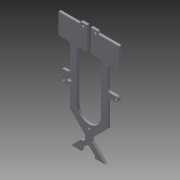
# Autodesk Inventor part: dissipador curvas 2mm v2
Saved by Autodesk Inventor 2013 (Build 170138000, 138)
## iProperties
Created: 2015-01-15
Part Number: dissipador curvas 2mm v2
Material: Genérico
Document SubType Name: Modeling
Designer: fernando.santanna
Density: 1 g/cm^3
Author: fernando.santanna
Autodesk Inventor part; units mm, degrees
ref_plane "YZ Plane" through (0, 0, 0) normal (1, 0, 0) x (0, 1, 0)
ref_plane "XZ Plane" through (0, 0, 0) normal (0, 1, 0) x (-1, 0, 0)
sketch "Bloco2" plane through (0, 0, 0) normal (0, 0, 1) x (1, 0, 0)
  line L0 (61.8192, 99.9321) -> (61.8192, 104.9321) construction
  line L1 (61.8192, 104.9321) -> (61.8192, 99.9321)
  line L2 (57.3192, 104.9321) -> (58.3192, 104.9321)
  line L3 (58.3192, 104.9321) -> (58.3192, 99.9321)
  line L4 (58.3192, 99.9321) -> (57.3192, 99.9321)
  line L5 (57.3192, 99.9321) -> (57.3192, 104.9321)
  line L6 (65.3192, 104.9321) -> (66.3192, 104.9321)
  line L7 (66.3192, 104.9321) -> (66.3192, 99.9321)
  line L8 (66.3192, 99.9321) -> (65.3192, 99.9321)
  line L9 (65.3192, 99.9321) -> (65.3192, 104.9321)
  point P0 (61.8192, 102.4321)
  dimension "d1" = 1
  dimension "d3" = 3.5
  dimension "d4" = 5
  dimension "d5" = 1
  dimension "d6" = 5
  dimension "d7" = 3.5
  measures "d1" distance of L3.end L4.end
  measures "d3" distance between parallel lines of L0 L3
  measures "d4" distance of L4.end L2.start
  measures "d5" distance of L7.end L8.end
  measures "d6" distance of L6.end L7.end
  measures "d7" distance between parallel lines of L1 L9
sketch "Bloco1" plane through (0, 0, 0) normal (0, 0, 1) x (1, 0, 0)
  arc A0 (51.7292, 104.9321) -> (48.7292, 101.9321) centre (51.7292, 101.9321) ccw construction
  arc A1 (93.7292, 2.9321) -> (91.7292, 4.9321) centre (91.7292, 2.9321) ccw construction
  line L0 (64.3092, -0.0679) -> (64.3092, 4.9321) construction
  circle A2 centre (73.7292, 25.9321) radius 1.1 construction
  circle A3 centre (51.5292, 57.9321) radius 1.1 construction
  circle A4 centre (94.7292, 50.4321) radius 1.1 construction
  circle A5 centre (56.5292, 2.9321) radius 1.1 construction
  circle A6 centre (68.7292, 96.9321) radius 1.1 construction
  circle A7 centre (91.7292, 2.9321) radius 1.1 construction
  circle A8 centre (78.7292, 96.9321) radius 1.1 construction
  arc A9 (91.2292, 48.4321) -> (89.2292, 46.4321) centre (91.2292, 46.4321) ccw construction
  line L1 (91.2292, 48.4321) -> (94.7807, 48.4321) construction
  arc A10 (94.7292, 48.4321) -> (96.7292, 50.4321) centre (94.7292, 50.4321) ccw construction
  line L2 (96.7292, 50.3807) -> (96.7292, 53.9321) construction
  arc A11 (91.1261, 55.1256) -> (90.851, 51.4175) centre (90.2532, 53.3261) ccw construction
  arc A12 (96.7292, 53.9321) -> (94.7292, 55.9321) centre (94.7292, 53.9321) ccw construction
  line L3 (91.2292, 55.9321) -> (94.7292, 55.9321) construction
  arc A13 (89.2292, 57.9321) -> (91.2292, 55.9321) centre (91.2292, 57.9321) ccw construction
  line L4 (83.7292, 38.9321) -> (83.7292, 77.9321) construction
  arc A14 (83.7292, 77.9321) -> (81.7292, 79.9321) centre (81.7292, 77.9321) ccw construction
  line L5 (77.2292, 79.9321) -> (81.7292, 79.9321) construction
  arc A15 (75.2292, 81.9321) -> (77.2292, 79.9321) centre (77.2292, 81.9321) ccw construction
  arc A16 (91.3396, 79.9321) -> (89.2292, 77.9352) centre (91.2292, 77.9352) ccw construction
  line L6 (91.3396, 79.9321) -> (96.8396, 79.9321) construction
  arc A17 (96.8396, 79.9321) -> (98.8396, 81.9321) centre (96.8396, 81.9321) ccw construction
  arc A18 (98.8396, 102.078) -> (95.9854, 104.9321) centre (95.9854, 102.078) ccw construction
  line L7 (63.7292, 38.9321) -> (63.7292, 76.9321) construction
  line L8 (48.7292, 81.9321) -> (48.7292, 101.9321) construction
  line L9 (72.2292, 81.9321) -> (72.2292, 101.9321) construction
  arc A19 (72.2292, 101.9321) -> (69.2292, 104.9321) centre (69.2292, 101.9321) ccw construction
  line L10 (84.2992, -0.0679) -> (84.2992, 4.9321) construction
  arc A20 (78.2292, 104.9321) -> (75.2292, 101.9321) centre (78.2292, 101.9321) ccw construction
  line L11 (86.8092, 101.8901) -> (86.8092, 104.9321) construction
  line L12 (78.2292, 104.9321) -> (95.9854, 104.9321) construction
  line L13 (89.2292, 57.9321) -> (89.2292, 77.9352) construction
  circle A21 centre (90.2532, 53.3261) radius 2 construction
  line L14 (83.7292, 38.9321) -> (83.7292, 76.9321) construction
  line L15 (51.7292, 104.9321) -> (69.2292, 104.9321) construction
  arc A22 (70.2292, 79.9321) -> (72.2292, 81.9321) centre (70.2292, 81.9321) ccw construction
  arc A23 (48.7292, 81.9321) -> (50.7292, 79.9321) centre (50.7292, 81.9321) ccw construction
  line L16 (50.7292, 79.9321) -> (56.2292, 79.9321) construction
  arc A24 (58.2292, 77.9321) -> (56.2292, 79.9321) centre (56.2292, 77.9321) ccw construction
  line L17 (65.7292, 79.9321) -> (70.2292, 79.9321) construction
  arc A25 (65.7292, 79.9321) -> (63.7292, 77.9321) centre (65.7292, 77.9321) ccw construction
  line L18 (58.2292, 72.4321) -> (58.2292, 77.9321) construction
  line L19 (63.7292, 38.9321) -> (63.7292, 77.9321) construction
  arc A26 (56.2292, 59.9321) -> (58.2292, 61.9321) centre (56.2292, 61.9321) ccw construction
  line L20 (51.5292, 59.9321) -> (56.2292, 59.9321) construction
  arc A27 (51.5292, 59.9321) -> (51.5292, 55.9321) centre (51.5292, 57.9321) ccw construction
  line L21 (58.2292, 61.9321) -> (58.2292, 72.4321) construction
  line L22 (51.5292, 55.9321) -> (56.2292, 55.9321) construction
  arc A28 (58.2292, 53.9321) -> (56.2292, 55.9321) centre (56.2292, 53.9321) ccw construction
  line L23 (58.2292, 33.2606) -> (58.2292, 53.9321) construction
  arc A29 (63.7292, 38.9321) -> (73.7292, 28.9321) centre (73.7292, 38.9321) ccw construction
  line L24 (58.2292, 33.2606) -> (71.1434, 20.3463) construction
  arc A30 (73.7292, 28.9321) -> (83.7292, 38.9321) centre (73.7292, 38.9321) ccw construction
  arc A31 (71.1434, 17.5179) -> (71.1434, 20.3463) centre (69.7292, 18.9321) ccw construction
  line L25 (58.5577, 4.9321) -> (71.1434, 17.5179) construction
  line L26 (56.5292, 4.9321) -> (58.5434, 4.9321) construction
  arc A32 (56.5292, 4.9321) -> (54.5292, 2.9321) centre (56.5292, 2.9321) ccw construction
  line L27 (54.5292, -0.0679) -> (54.5292, 2.9321) construction
  line L28 (68.5592, -0.0679) -> (68.5592, 8.5826) construction
  line L29 (68.5592, 8.5826) -> (72.819, 12.8424) construction
  arc A33 (75.6394, 12.8424) -> (72.819, 12.8424) centre (74.2292, 11.4321) ccw construction
  line L30 (75.6394, 12.8424) -> (80.0492, 8.4326) construction
  line L31 (80.0492, -0.0679) -> (80.0492, 8.4326) construction
  line L32 (93.7292, -0.0679) -> (93.7292, 2.9321) construction
  line L33 (89.9008, 4.9321) -> (91.7292, 4.9321) construction
  line L34 (77.315, 17.5179) -> (89.9008, 4.9321) construction
  line L35 (77.315, 20.3463) -> (89.2292, 32.2606) construction
  arc A34 (77.315, 20.3463) -> (77.315, 17.5179) centre (78.7292, 18.9321) ccw construction
  line L36 (89.2292, 32.2606) -> (89.2292, 46.4321) construction
  line L37 (75.2292, 81.9321) -> (75.2292, 101.9321) construction
  line L38 (98.8396, 81.9321) -> (98.8396, 102.078) construction
  line L39 (54.5292, -0.0679) -> (68.5592, -0.0679) construction
  line L40 (80.0492, -0.0679) -> (93.7292, -0.0679) construction
  line L41 (61.8192, 99.9321) -> (61.8192, 104.9321) construction
  line L42 (61.8192, 104.9321) -> (61.8192, 99.9321)
  line L43 (57.3192, 104.9321) -> (58.3192, 104.9321)
  line L44 (58.3192, 104.9321) -> (58.3192, 99.9321)
  line L45 (58.3192, 99.9321) -> (57.3192, 99.9321)
  line L46 (57.3192, 99.9321) -> (57.3192, 104.9321)
  line L47 (65.3192, 104.9321) -> (66.3192, 104.9321)
  line L48 (66.3192, 104.9321) -> (66.3192, 99.9321)
  line L49 (66.3192, 99.9321) -> (65.3192, 99.9321)
  line L50 (65.3192, 99.9321) -> (65.3192, 104.9321)
  line L51 (86.8092, 99.9321) -> (86.8092, 104.9321) construction
  line L52 (86.8092, 104.9321) -> (86.8092, 99.9321)
  line L53 (82.3092, 104.9321) -> (83.3092, 104.9321)
  line L54 (83.3092, 104.9321) -> (83.3092, 99.9321)
  line L55 (83.3092, 99.9321) -> (82.3092, 99.9321)
  line L56 (82.3092, 99.9321) -> (82.3092, 104.9321)
  line L57 (90.3092, 104.9321) -> (91.3092, 104.9321)
  line L58 (91.3092, 104.9321) -> (91.3092, 99.9321)
  line L59 (91.3092, 99.9321) -> (90.3092, 99.9321)
  line L60 (90.3092, 99.9321) -> (90.3092, 104.9321)
  line L61 (84.2992, -0.0679) -> (84.2992, 4.9321) construction
  line L62 (84.2992, 4.9321) -> (84.2992, -0.0679)
  line L63 (79.7992, 4.9321) -> (80.7992, 4.9321)
  line L64 (80.7992, 4.9321) -> (80.7992, -0.0679)
  line L65 (80.7992, -0.0679) -> (79.7992, -0.0679)
  line L66 (79.7992, -0.0679) -> (79.7992, 4.9321)
  line L67 (87.7992, 4.9321) -> (88.7992, 4.9321)
  line L68 (88.7992, 4.9321) -> (88.7992, -0.0679)
  line L69 (88.7992, -0.0679) -> (87.7992, -0.0679)
  line L70 (87.7992, -0.0679) -> (87.7992, 4.9321)
  line L71 (64.3092, -0.0679) -> (64.3092, 4.9321) construction
  line L72 (64.3092, 4.9321) -> (64.3092, -0.0679)
  line L73 (59.8092, 4.9321) -> (60.8092, 4.9321)
  line L74 (60.8092, 4.9321) -> (60.8092, -0.0679)
  line L75 (60.8092, -0.0679) -> (59.8092, -0.0679)
  line L76 (59.8092, -0.0679) -> (59.8092, 4.9321)
  line L77 (67.8092, 4.9321) -> (68.8092, 4.9321)
  line L78 (68.8092, 4.9321) -> (68.8092, -0.0679)
  line L79 (68.8092, -0.0679) -> (67.8092, -0.0679)
  line L80 (67.8092, -0.0679) -> (67.8092, 4.9321)
  point P0 (27.7161, 5.6229)
sketch "Esboço2" plane through (0, 0, 0) normal (0, 1, 0) x (-1, 0, 0)
  arc A0 (-62.8439, 117.7004) -> (-65.8439, 114.7004) centre (-62.8439, 114.7004) ccw construction
  arc A1 (-20.8439, 15.7004) -> (-22.8439, 17.7004) centre (-22.8439, 15.7004) ccw construction
  line L0 (-50.2639, 12.7004) -> (-50.2639, 17.7004) construction
  circle A2 centre (-40.8439, 38.7004) radius 1.1 construction
  circle A3 centre (-63.0439, 70.7004) radius 1.1 construction
  circle A4 centre (-19.8439, 63.2004) radius 1.1 construction
  circle A5 centre (-58.0439, 15.7004) radius 1.1 construction
  circle A6 centre (-45.8439, 109.7004) radius 1.1 construction
  circle A7 centre (-22.8439, 15.7004) radius 1.1 construction
  circle A8 centre (-35.8439, 109.7004) radius 1.1 construction
  arc A9 (-23.3439, 61.2004) -> (-25.3439, 59.2004) centre (-23.3439, 59.2004) ccw construction
  line L1 (-23.3439, 61.2004) -> (-19.7924, 61.2004) construction
  arc A10 (-19.8439, 61.2004) -> (-17.8439, 63.2004) centre (-19.8439, 63.2004) ccw construction
  line L2 (-17.8439, 63.1489) -> (-17.8439, 66.7004) construction
  arc A11 (-23.4471, 67.8939) -> (-23.7222, 64.1858) centre (-24.3199, 66.0944) ccw construction
  arc A12 (-17.8439, 66.7004) -> (-19.8439, 68.7004) centre (-19.8439, 66.7004) ccw construction
  line L3 (-23.3439, 68.7004) -> (-19.8439, 68.7004) construction
  arc A13 (-25.3439, 70.7004) -> (-23.3439, 68.7004) centre (-23.3439, 70.7004) ccw construction
  line L4 (-30.8439, 51.7004) -> (-30.8439, 90.7004) construction
  arc A14 (-30.8439, 90.7004) -> (-32.8439, 92.7004) centre (-32.8439, 90.7004) ccw construction
  line L5 (-37.3439, 92.7004) -> (-32.8439, 92.7004) construction
  arc A15 (-39.3439, 94.7004) -> (-37.3439, 92.7004) centre (-37.3439, 94.7004) ccw construction
  arc A16 (-23.2335, 92.7004) -> (-25.3439, 90.7034) centre (-23.3439, 90.7034) ccw construction
  line L6 (-23.2335, 92.7004) -> (-17.7335, 92.7004) construction
  arc A17 (-17.7335, 92.7004) -> (-15.7335, 94.7004) centre (-17.7335, 94.7004) ccw construction
  arc A18 (-15.7335, 114.8462) -> (-18.5877, 117.7004) centre (-18.5877, 114.8462) ccw construction
  line L7 (-50.8439, 51.7004) -> (-50.8439, 89.7004) construction
  line L8 (-65.8439, 94.7004) -> (-65.8439, 114.7004) construction
  line L9 (-42.3439, 94.7004) -> (-42.3439, 114.7004) construction
  arc A19 (-42.3439, 114.7004) -> (-45.3439, 117.7004) centre (-45.3439, 114.7004) ccw construction
  line L10 (-30.2739, 12.7004) -> (-30.2739, 17.7004) construction
  arc A20 (-36.3439, 117.7004) -> (-39.3439, 114.7004) centre (-36.3439, 114.7004) ccw construction
  line L11 (-27.7639, 114.6583) -> (-27.7639, 117.7004) construction
  line L12 (-36.3439, 117.7004) -> (-18.5877, 117.7004) construction
  line L13 (-25.3439, 70.7004) -> (-25.3439, 90.7034) construction
  circle A21 centre (-24.3199, 66.0944) radius 2 construction
  line L14 (-30.8439, 51.7004) -> (-30.8439, 89.7004) construction
  line L15 (-62.8439, 117.7004) -> (-45.3439, 117.7004) construction
  arc A22 (-44.3439, 92.7004) -> (-42.3439, 94.7004) centre (-44.3439, 94.7004) ccw construction
  arc A23 (-65.8439, 94.7004) -> (-63.8439, 92.7004) centre (-63.8439, 94.7004) ccw construction
  line L16 (-63.8439, 92.7004) -> (-58.3439, 92.7004) construction
  arc A24 (-56.3439, 90.7004) -> (-58.3439, 92.7004) centre (-58.3439, 90.7004) ccw construction
  line L17 (-48.8439, 92.7004) -> (-44.3439, 92.7004) construction
  arc A25 (-48.8439, 92.7004) -> (-50.8439, 90.7004) centre (-48.8439, 90.7004) ccw construction
  line L18 (-56.3439, 85.2004) -> (-56.3439, 90.7004) construction
  line L19 (-50.8439, 51.7004) -> (-50.8439, 90.7004) construction
  arc A26 (-58.3439, 72.7004) -> (-56.3439, 74.7004) centre (-58.3439, 74.7004) ccw construction
  line L20 (-63.0439, 72.7004) -> (-58.3439, 72.7004) construction
  arc A27 (-63.0439, 72.7004) -> (-63.0439, 68.7004) centre (-63.0439, 70.7004) ccw construction
  line L21 (-56.3439, 74.7004) -> (-56.3439, 85.2004) construction
  line L22 (-63.0439, 68.7004) -> (-58.3439, 68.7004) construction
  arc A28 (-56.3439, 66.7004) -> (-58.3439, 68.7004) centre (-58.3439, 66.7004) ccw construction
  line L23 (-56.3439, 46.0288) -> (-56.3439, 66.7004) construction
  arc A29 (-50.8439, 51.7004) -> (-40.8439, 41.7004) centre (-40.8439, 51.7004) ccw construction
  line L24 (-56.3439, 46.0288) -> (-43.4297, 33.1146) construction
  arc A30 (-40.8439, 41.7004) -> (-30.8439, 51.7004) centre (-40.8439, 51.7004) ccw construction
  arc A31 (-43.4297, 30.2862) -> (-43.4297, 33.1146) centre (-44.8439, 31.7004) ccw construction
  line L25 (-56.0155, 17.7004) -> (-43.4297, 30.2862) construction
  line L26 (-58.0439, 17.7004) -> (-56.0297, 17.7004) construction
  arc A32 (-58.0439, 17.7004) -> (-60.0439, 15.7004) centre (-58.0439, 15.7004) ccw construction
  line L27 (-60.0439, 12.7004) -> (-60.0439, 15.7004) construction
  line L28 (-46.0139, 12.7004) -> (-46.0139, 21.3508) construction
  line L29 (-46.0139, 21.3508) -> (-41.7541, 25.6106) construction
  arc A33 (-38.9337, 25.6106) -> (-41.7541, 25.6106) centre (-40.3439, 24.2004) ccw construction
  line L30 (-38.9337, 25.6106) -> (-34.5239, 21.2008) construction
  line L31 (-34.5239, 12.7004) -> (-34.5239, 21.2008) construction
  line L32 (-20.8439, 12.7004) -> (-20.8439, 15.7004) construction
  line L33 (-24.6723, 17.7004) -> (-22.8439, 17.7004) construction
  line L34 (-37.2581, 30.2862) -> (-24.6723, 17.7004) construction
  line L35 (-37.2581, 33.1146) -> (-25.3439, 45.0288) construction
  arc A34 (-37.2581, 33.1146) -> (-37.2581, 30.2862) centre (-35.8439, 31.7004) ccw construction
  line L36 (-25.3439, 45.0288) -> (-25.3439, 59.2004) construction
  line L37 (-39.3439, 94.7004) -> (-39.3439, 114.7004) construction
  line L38 (-15.7335, 94.7004) -> (-15.7335, 114.8462) construction
  line L39 (-60.0439, 12.7004) -> (-46.0139, 12.7004) construction
  line L40 (-34.5239, 12.7004) -> (-20.8439, 12.7004) construction
  line L41 (-52.7539, 112.7004) -> (-52.7539, 117.7004) construction
  line L42 (-52.7539, 117.7004) -> (-52.7539, 112.7004)
  line L43 (-57.2539, 117.7004) -> (-56.2539, 117.7004)
  line L44 (-56.2539, 117.7004) -> (-56.2539, 112.7004)
  line L45 (-56.2539, 112.7004) -> (-57.2539, 112.7004)
  line L46 (-57.2539, 112.7004) -> (-57.2539, 117.7004)
  line L47 (-49.2539, 117.7004) -> (-48.2539, 117.7004)
  line L48 (-48.2539, 117.7004) -> (-48.2539, 112.7004)
  line L49 (-48.2539, 112.7004) -> (-49.2539, 112.7004)
  line L50 (-49.2539, 112.7004) -> (-49.2539, 117.7004)
  line L51 (-27.7639, 112.7004) -> (-27.7639, 117.7004) construction
  line L52 (-27.7639, 117.7004) -> (-27.7639, 112.7004)
  line L53 (-32.2639, 117.7004) -> (-31.2639, 117.7004)
  line L54 (-31.2639, 117.7004) -> (-31.2639, 112.7004)
  line L55 (-31.2639, 112.7004) -> (-32.2639, 112.7004)
  line L56 (-32.2639, 112.7004) -> (-32.2639, 117.7004)
  line L57 (-24.2639, 117.7004) -> (-23.2639, 117.7004)
  line L58 (-23.2639, 117.7004) -> (-23.2639, 112.7004)
  line L59 (-23.2639, 112.7004) -> (-24.2639, 112.7004)
  line L60 (-24.2639, 112.7004) -> (-24.2639, 117.7004)
  line L61 (-30.2739, 12.7004) -> (-30.2739, 17.7004) construction
  line L62 (-30.2739, 17.7004) -> (-30.2739, 12.7004)
  line L63 (-34.7739, 17.7004) -> (-33.7739, 17.7004)
  line L64 (-33.7739, 17.7004) -> (-33.7739, 12.7004)
  line L65 (-33.7739, 12.7004) -> (-34.7739, 12.7004)
  line L66 (-34.7739, 12.7004) -> (-34.7739, 17.7004)
  line L67 (-26.7739, 17.7004) -> (-25.7739, 17.7004)
  line L68 (-25.7739, 17.7004) -> (-25.7739, 12.7004)
  line L69 (-25.7739, 12.7004) -> (-26.7739, 12.7004)
  line L70 (-26.7739, 12.7004) -> (-26.7739, 17.7004)
  line L71 (-50.2639, 12.7004) -> (-50.2639, 17.7004) construction
  line L72 (-50.2639, 17.7004) -> (-50.2639, 12.7004)
  line L73 (-54.7639, 17.7004) -> (-53.7639, 17.7004)
  line L74 (-53.7639, 17.7004) -> (-53.7639, 12.7004)
  line L75 (-53.7639, 12.7004) -> (-54.7639, 12.7004)
  line L76 (-54.7639, 12.7004) -> (-54.7639, 17.7004)
  line L77 (-46.7639, 17.7004) -> (-45.7639, 17.7004)
  line L78 (-45.7639, 17.7004) -> (-45.7639, 12.7004)
  line L79 (-45.7639, 12.7004) -> (-46.7639, 12.7004)
  line L80 (-46.7639, 12.7004) -> (-46.7639, 17.7004)
  point P0 (0, 0)
sketch "Esboço3" plane through (0, 0, 0) normal (0, 1, 0) x (-1, 0, 0)
  line L0 (-62.8439, 117.7004) -> (-45.3439, 117.7004) construction
  arc A0 (-62.8439, 117.7004) -> (-65.8439, 114.7004) centre (-62.8439, 114.7004) ccw construction
  line L1 (-65.8439, 94.7004) -> (-65.8439, 114.7004) construction
  arc A1 (-42.3439, 114.7004) -> (-45.3439, 117.7004) centre (-45.3439, 114.7004) ccw construction
  line L2 (-42.3439, 94.7004) -> (-42.3439, 114.7004) construction
  line L3 (-39.3439, 94.7004) -> (-39.3439, 114.7004) construction
  arc A2 (-36.3439, 117.7004) -> (-39.3439, 114.7004) centre (-36.3439, 114.7004) ccw construction
  line L4 (-36.3439, 117.7004) -> (-18.5877, 117.7004) construction
  circle A3 centre (-35.8439, 109.7004) radius 1.1 construction
  line L5 (-15.7335, 94.7004) -> (-15.7335, 114.8462) construction
  arc A4 (-15.7335, 114.8462) -> (-18.5877, 117.7004) centre (-18.5877, 114.8462) ccw construction
  line L6 (-37.3439, 92.7004) -> (-32.8439, 92.7004) construction
  arc A5 (-39.3439, 94.7004) -> (-37.3439, 92.7004) centre (-37.3439, 94.7004) ccw construction
  arc A6 (-30.8439, 90.7004) -> (-32.8439, 92.7004) centre (-32.8439, 90.7004) ccw construction
  arc A7 (-23.2335, 92.7004) -> (-25.3439, 90.7034) centre (-23.3439, 90.7034) ccw construction
  line L7 (-23.2335, 92.7004) -> (-17.7335, 92.7004) construction
  arc A8 (-17.7335, 92.7004) -> (-15.7335, 94.7004) centre (-17.7335, 94.7004) ccw construction
  arc A9 (-44.3439, 92.7004) -> (-42.3439, 94.7004) centre (-44.3439, 94.7004) ccw construction
  line L8 (-48.8439, 92.7004) -> (-44.3439, 92.7004) construction
  arc A10 (-48.8439, 92.7004) -> (-50.8439, 90.7004) centre (-48.8439, 90.7004) ccw construction
  arc A11 (-56.3439, 90.7004) -> (-58.3439, 92.7004) centre (-58.3439, 90.7004) ccw construction
  line L9 (-63.8439, 92.7004) -> (-58.3439, 92.7004) construction
  arc A12 (-65.8439, 94.7004) -> (-63.8439, 92.7004) centre (-63.8439, 94.7004) ccw construction
  line L10 (-56.3439, 85.2004) -> (-56.3439, 90.7004) construction
  line L11 (-50.8439, 51.7004) -> (-50.8439, 90.7004) construction
  line L12 (-56.3439, 74.7004) -> (-56.3439, 85.2004) construction
  line L13 (-30.8439, 51.7004) -> (-30.8439, 89.7004) construction
  line L14 (-30.8439, 51.7004) -> (-30.8439, 90.7004) construction
  arc A13 (-58.3439, 72.7004) -> (-56.3439, 74.7004) centre (-58.3439, 74.7004) ccw construction
  line L15 (-63.0439, 72.7004) -> (-58.3439, 72.7004) construction
  arc A14 (-63.0439, 72.7004) -> (-63.0439, 68.7004) centre (-63.0439, 70.7004) ccw construction
  line L16 (-63.0439, 68.7004) -> (-58.3439, 68.7004) construction
  arc A15 (-56.3439, 66.7004) -> (-58.3439, 68.7004) centre (-58.3439, 66.7004) ccw construction
  line L17 (-56.3439, 46.0288) -> (-56.3439, 66.7004) construction
  line L18 (-17.8439, 63.1489) -> (-17.8439, 66.7004) construction
  line L19 (-23.3439, 61.2004) -> (-19.7924, 61.2004) construction
  arc A16 (-19.8439, 61.2004) -> (-17.8439, 63.2004) centre (-19.8439, 63.2004) ccw construction
  arc A17 (-23.3439, 61.2004) -> (-25.3439, 59.2004) centre (-23.3439, 59.2004) ccw construction
  line L20 (-25.3439, 45.0288) -> (-25.3439, 59.2004) construction
  arc A18 (-40.8439, 41.7004) -> (-30.8439, 51.7004) centre (-40.8439, 51.7004) ccw construction
  arc A19 (-50.8439, 51.7004) -> (-40.8439, 41.7004) centre (-40.8439, 51.7004) ccw construction
  line L21 (-37.2581, 33.1146) -> (-25.3439, 45.0288) construction
  line L22 (-56.3439, 46.0288) -> (-43.4297, 33.1146) construction
  arc A20 (-43.4297, 30.2862) -> (-43.4297, 33.1146) centre (-44.8439, 31.7004) ccw construction
  arc A21 (-37.2581, 33.1146) -> (-37.2581, 30.2862) centre (-35.8439, 31.7004) ccw construction
  line L23 (-56.0155, 17.7004) -> (-43.4297, 30.2862) construction
  line L24 (-37.2581, 30.2862) -> (-24.6723, 17.7004) construction
  line L25 (-34.5239, 12.7004) -> (-34.5239, 21.2008) construction
  line L26 (-38.9337, 25.6106) -> (-34.5239, 21.2008) construction
  arc A22 (-38.9337, 25.6106) -> (-41.7541, 25.6106) centre (-40.3439, 24.2004) ccw construction
  line L27 (-46.0139, 21.3508) -> (-41.7541, 25.6106) construction
  line L28 (-46.0139, 12.7004) -> (-46.0139, 21.3508) construction
  line L29 (-58.0439, 17.7004) -> (-56.0297, 17.7004) construction
  arc A23 (-58.0439, 17.7004) -> (-60.0439, 15.7004) centre (-58.0439, 15.7004) ccw construction
  line L30 (-60.0439, 12.7004) -> (-60.0439, 15.7004) construction
  line L31 (-60.0439, 12.7004) -> (-46.0139, 12.7004) construction
  line L32 (-34.5239, 12.7004) -> (-20.8439, 12.7004) construction
  line L33 (-20.8439, 12.7004) -> (-20.8439, 15.7004) construction
  arc A24 (-20.8439, 15.7004) -> (-22.8439, 17.7004) centre (-22.8439, 15.7004) ccw construction
  line L34 (-24.6723, 17.7004) -> (-22.8439, 17.7004) construction
  line L35 (-62.8439, 117.7004) -> (-45.3439, 117.7004)
  line L36 (-42.3439, 114.7004) -> (-42.3439, 94.7004)
  line L37 (-65.8439, 114.7004) -> (-65.8439, 94.7004)
  line L38 (-63.8439, 92.7004) -> (-58.3439, 92.7004)
  line L39 (-48.8439, 92.7004) -> (-44.3439, 92.7004)
  line L40 (-56.3439, 90.7004) -> (-56.3439, 74.7004)
  line L41 (-50.8439, 90.7004) -> (-50.8439, 51.7004)
  line L42 (-56.3439, 66.7004) -> (-56.3439, 46.0288)
  line L43 (-58.3439, 72.7004) -> (-63.0439, 72.7004)
  line L44 (-58.3439, 68.7004) -> (-63.0439, 68.7004)
  line L45 (-39.3439, 114.7004) -> (-39.3439, 94.7004)
  line L46 (-37.3439, 92.7004) -> (-32.8439, 92.7004)
  line L47 (-36.3439, 117.7004) -> (-18.5877, 117.7004)
  line L48 (-15.7335, 114.8462) -> (-15.7335, 94.7004)
  line L49 (-17.7335, 92.7004) -> (-23.2335, 92.7004)
  line L50 (-30.8439, 90.7004) -> (-30.8439, 51.7004)
  line L51 (-17.8439, 66.7004) -> (-17.8439, 63.2004)
  line L52 (-19.8439, 61.2004) -> (-23.3439, 61.2004)
  line L53 (-25.3439, 59.2004) -> (-25.3439, 45.0288)
  line L54 (-25.3439, 45.0288) -> (-37.2581, 33.1146)
  line L55 (-56.3439, 46.0288) -> (-43.4297, 33.1146)
  line L56 (-43.4297, 30.2862) -> (-56.0297, 17.7004)
  line L57 (-37.2581, 30.2862) -> (-24.6723, 17.7004)
  line L58 (-46.0139, 21.3508) -> (-41.7541, 25.6106)
  line L59 (-38.9337, 25.6106) -> (-34.5239, 21.2008)
  line L60 (-46.0139, 21.3508) -> (-46.0139, 17.7004)
  line L61 (-34.5239, 21.2008) -> (-34.5239, 17.7004)
  arc A25 (-42.3439, 114.7004) -> (-45.3439, 117.7004) centre (-45.3439, 114.7004) ccw
  arc A26 (-36.3439, 117.7004) -> (-39.3439, 114.7004) centre (-36.3439, 114.7004) ccw
  arc A27 (-15.7335, 114.8462) -> (-18.5877, 117.7004) centre (-18.5877, 114.8462) ccw
  arc A28 (-17.7335, 92.7004) -> (-15.7335, 94.7004) centre (-17.7335, 94.7004) ccw
  arc A29 (-23.2335, 92.7004) -> (-25.3439, 90.7034) centre (-23.3439, 90.7034) ccw
  arc A30 (-30.8439, 90.7004) -> (-32.8439, 92.7004) centre (-32.8439, 90.7004) ccw
  arc A31 (-39.3439, 94.7004) -> (-37.3439, 92.7004) centre (-37.3439, 94.7004) ccw
  arc A32 (-44.3439, 92.7004) -> (-42.3439, 94.7004) centre (-44.3439, 94.7004) ccw
  arc A33 (-48.8439, 92.7004) -> (-50.8439, 90.7004) centre (-48.8439, 90.7004) ccw
  arc A34 (-65.8439, 94.7004) -> (-63.8439, 92.7004) centre (-63.8439, 94.7004) ccw
  arc A35 (-56.3439, 90.7004) -> (-58.3439, 92.7004) centre (-58.3439, 90.7004) ccw
  arc A36 (-58.3439, 72.7004) -> (-56.3439, 74.7004) centre (-58.3439, 74.7004) ccw
  arc A37 (-63.0439, 72.7004) -> (-63.0439, 68.7004) centre (-63.0439, 70.7004) ccw
  arc A38 (-56.3439, 66.7004) -> (-58.3439, 68.7004) centre (-58.3439, 66.7004) ccw
  arc A39 (-50.8439, 51.7004) -> (-30.8439, 51.7004) centre (-40.8439, 51.7004) ccw
  arc A40 (-19.8439, 61.2004) -> (-17.8439, 63.2004) centre (-19.8439, 63.2004) ccw
  arc A41 (-23.3439, 61.2004) -> (-25.3439, 59.2004) centre (-23.3439, 59.2004) ccw
  arc A42 (-43.4297, 30.2862) -> (-43.4297, 33.1146) centre (-44.8439, 31.7004) ccw
  arc A43 (-37.2581, 33.1146) -> (-37.2581, 30.2862) centre (-35.8439, 31.7004) ccw
  arc A44 (-38.9337, 25.6106) -> (-41.7541, 25.6106) centre (-40.3439, 24.2004) ccw
  arc A45 (-62.8439, 117.7004) -> (-65.8439, 114.7004) centre (-62.8439, 114.7004) ccw
  line L62 (-46.0139, 19.5256) -> (-54.2024, 19.5256)
  line L63 (-34.5239, 19.4506) -> (-26.4226, 19.4506)
  circle A46 centre (-63.0439, 70.7004) radius 1.1
  circle A47 centre (-24.3199, 66.0944) radius 2.2
  circle A48 centre (-19.8439, 63.2004) radius 1.1
  circle A49 centre (-35.8439, 109.7004) radius 1.1
  circle A50 centre (-45.8439, 109.7004) radius 1.1
  circle A51 centre (-40.8439, 38.7004) radius 1.1
  line L64 (-17.8439, 66.7004) -> (-17.8439, 68.5102)
  line L65 (-20.003, 70.6692) -> (-22.8176, 70.6692)
  arc A52 (-17.8439, 68.5102) -> (-20.003, 70.6692) centre (-20.003, 68.5102) ccw
  arc A53 (-25.3439, 73.1956) -> (-22.8176, 70.6692) centre (-22.8176, 73.1956) ccw
  line L66 (-25.3439, 73.1956) -> (-25.3439, 90.7034)
  line L67 (-15.7335, 109.8073) -> (-32.6508, 109.8073)
  arc A54 (-33.3637, 110.5201) -> (-32.6508, 109.8073) centre (-32.6508, 110.5201) ccw
  arc A55 (-33.3637, 110.5201) -> (-34.5439, 111.7004) centre (-34.5439, 110.5201) ccw
  line L68 (-34.5439, 111.7004) -> (-39.3439, 111.7004)
  line L69 (-48.2539, 117.7004) -> (-48.2539, 112.7004) projected
  line L70 (-65.8439, 109.8073) -> (-49.037, 109.8073)
  arc A56 (-49.037, 109.8073) -> (-48.3242, 110.5201) centre (-49.037, 110.5201) ccw
  arc A57 (-47.1439, 111.7004) -> (-48.3242, 110.5201) centre (-47.1439, 110.5201) ccw
  line L71 (-47.1439, 111.7004) -> (-42.3439, 111.7004)
  point P0 (-25.3439, 70.7004)
  point P1 (-63.0439, 70.7004)
  point P2 (-19.8439, 68.7004)
  point P3 (-23.3439, 68.7004)
  point P4 (-22.8439, 15.7004)
  dimension "d8" = 2.2
  dimension "d9" = 4.4
  dimension "d10" = 2.2
  dimension "d11" = 2.2
  dimension "d12" = 2.2
  dimension "d13" = 2.2
  dimension "d23" = 6
  dimension "d25" = 1.3
  constraints: 84 tangent, 72 end point, 54 point on circle, 33 centre point, 18 collinear, 10 point on line, 8 perpendicular, 6 coincident, 3 parallel, 2 midpoint, 1 concentric, 1 horizontal alignment
  measures "d8" diameter of A46
  measures "d9" diameter of A47
  measures "d10" diameter of A48
  measures "d11" diameter of A49
  measures "d12" diameter of A50
  measures "d13" diameter of A51
  measures "d23" distance from line of L4.start L68
  measures "d25" horizontal distance of L68.start A3.centre
extrude "Extrusão3" add sketch "Esboço3" along normal blind 2 contours L70 A56 A57 L71 L36 A32 L39 A33 L41 A39 L50 A30 L46 A31 L45 L68 A55 A54 L67 L48 A28 L49 A29 L66 A53 L65 A52 L64 L51 A40 L52 A41 L53 L54 A43 L57 L63 L61 L59 A44 L58 L60 L62 L56 A42 L55 L42 A38 L44 A37 L43 A36 L40 A35 L38 A34 L37
ref_plane "Plano de trabalho1" through (0, 2, 0) normal (0, 1, 0) x (1, 0, 0)
sketch "Esboço5" plane through (0, 0, 0) normal (0, -1, 0) x (1, 0, 0)
  circle A0 centre (24.3199, 66.0944) radius 2.2 projected
  circle A1 centre (40.8439, 38.7004) radius 1.1 projected
  circle A2 centre (45.8439, 109.7004) radius 1.1 projected
  circle A3 centre (35.8439, 109.7004) radius 1.1 projected
  circle A4 centre (19.8439, 63.2004) radius 1.1 projected
  circle A5 centre (63.0439, 70.7004) radius 1.1 projected
  arc A6 (63.8439, 92.7004) -> (65.8439, 94.7004) centre (63.8439, 94.7004) ccw projected
  line L0 (65.8439, 109.8073) -> (65.8439, 94.7004) projected
  line L1 (49.037, 109.8073) -> (65.8439, 109.8073) projected
  arc A7 (48.3242, 110.5201) -> (49.037, 109.8073) centre (49.037, 110.5201) ccw projected
  arc A8 (48.3242, 110.5201) -> (47.1439, 111.7004) centre (47.1439, 110.5201) ccw projected
  line L2 (42.3439, 111.7004) -> (47.1439, 111.7004) projected
  line L3 (42.3439, 94.7004) -> (42.3439, 111.7004) projected
  arc A9 (42.3439, 94.7004) -> (44.3439, 92.7004) centre (44.3439, 94.7004) ccw projected
  line L4 (48.8439, 92.7004) -> (44.3439, 92.7004) projected
  arc A10 (50.8439, 90.7004) -> (48.8439, 92.7004) centre (48.8439, 90.7004) ccw projected
  line L5 (50.8439, 51.7004) -> (50.8439, 90.7004) projected
  arc A11 (30.8439, 51.7004) -> (50.8439, 51.7004) centre (40.8439, 51.7004) ccw projected
  line L6 (30.8439, 90.7004) -> (30.8439, 51.7004) projected
  arc A12 (32.8439, 92.7004) -> (30.8439, 90.7004) centre (32.8439, 90.7004) ccw projected
  line L7 (37.3439, 92.7004) -> (32.8439, 92.7004) projected
  arc A13 (37.3439, 92.7004) -> (39.3439, 94.7004) centre (37.3439, 94.7004) ccw projected
  line L8 (39.3439, 111.7004) -> (39.3439, 94.7004) projected
  line L9 (34.5439, 111.7004) -> (39.3439, 111.7004) projected
  arc A14 (34.5439, 111.7004) -> (33.3637, 110.5201) centre (34.5439, 110.5201) ccw projected
  arc A15 (32.6508, 109.8073) -> (33.3637, 110.5201) centre (32.6508, 110.5201) ccw projected
  line L10 (15.7335, 109.8073) -> (32.6508, 109.8073) projected
  line L11 (15.7335, 94.7004) -> (15.7335, 109.8073) projected
  arc A16 (15.7335, 94.7004) -> (17.7335, 92.7004) centre (17.7335, 94.7004) ccw projected
  line L12 (23.2335, 92.7004) -> (17.7335, 92.7004) projected
  arc A17 (25.3439, 90.7034) -> (23.2335, 92.7004) centre (23.3439, 90.7034) ccw projected
  line L13 (25.3439, 73.1956) -> (25.3439, 90.7034) projected
  arc A18 (22.8176, 70.6692) -> (25.3439, 73.1956) centre (22.8176, 73.1956) ccw projected
  line L14 (20.003, 70.6692) -> (22.8176, 70.6692) projected
  arc A19 (20.003, 70.6692) -> (17.8439, 68.5102) centre (20.003, 68.5102) ccw projected
  line L15 (17.8439, 63.2004) -> (17.8439, 68.5102) projected
  arc A20 (17.8439, 63.2004) -> (19.8439, 61.2004) centre (19.8439, 63.2004) ccw projected
  line L16 (23.3439, 61.2004) -> (19.8439, 61.2004) projected
  arc A21 (25.3439, 59.2004) -> (23.3439, 61.2004) centre (23.3439, 59.2004) ccw projected
  line L17 (25.3439, 45.0288) -> (25.3439, 59.2004) projected
  line L18 (37.2581, 33.1146) -> (25.3439, 45.0288) projected
  arc A22 (37.2581, 30.2862) -> (37.2581, 33.1146) centre (35.8439, 31.7004) ccw projected
  line L19 (26.4226, 19.4506) -> (37.2581, 30.2862) projected
  line L20 (34.5239, 19.4506) -> (26.4226, 19.4506) projected
  line L21 (34.5239, 21.2008) -> (34.5239, 19.4506) projected
  line L22 (38.9337, 25.6106) -> (34.5239, 21.2008) projected
  arc A23 (41.7541, 25.6106) -> (38.9337, 25.6106) centre (40.3439, 24.2004) ccw projected
  line L23 (46.0139, 21.3508) -> (41.7541, 25.6106) projected
  line L24 (46.0139, 19.5256) -> (46.0139, 21.3508) projected
  line L25 (54.2024, 19.5256) -> (46.0139, 19.5256) projected
  line L26 (43.4297, 30.2862) -> (54.2024, 19.5256) projected
  arc A24 (43.4297, 33.1146) -> (43.4297, 30.2862) centre (44.8439, 31.7004) ccw projected
  line L27 (56.3439, 46.0288) -> (43.4297, 33.1146) projected
  line L28 (56.3439, 66.7004) -> (56.3439, 46.0288) projected
  arc A25 (58.3439, 68.7004) -> (56.3439, 66.7004) centre (58.3439, 66.7004) ccw projected
  line L29 (63.0439, 68.7004) -> (58.3439, 68.7004) projected
  arc A26 (63.0439, 68.7004) -> (63.0439, 72.7004) centre (63.0439, 70.7004) ccw projected
  line L30 (58.3439, 72.7004) -> (63.0439, 72.7004) projected
  arc A27 (56.3439, 74.7004) -> (58.3439, 72.7004) centre (58.3439, 74.7004) ccw projected
  line L31 (56.3439, 90.7004) -> (56.3439, 74.7004) projected
  arc A28 (58.3439, 92.7004) -> (56.3439, 90.7004) centre (58.3439, 90.7004) ccw projected
  line L32 (63.8439, 92.7004) -> (58.3439, 92.7004) projected
  point P0 (0, 0)
sketch "Esboço6" plane through (0, 0, 0) normal (0, -1, 0) x (1, 0, 0)
  line L0 (26.4226, 19.4506) -> (37.2581, 30.2862) projected
  circle A0 centre (35.8439, 28.8719) radius 1.5
  line L1 (37.2581, 33.1146) -> (25.3439, 45.0288) projected
  arc A1 (37.2581, 30.2862) -> (37.2581, 33.1146) centre (35.8439, 31.7004) ccw projected
  line L2 (63.8439, 92.7004) -> (58.3439, 92.7004) projected
  line L3 (35.8439, 27.3719) -> (34.3439, 27.3719)
  line L4 (34.3439, 28.8719) -> (34.3439, 27.3719)
  line L5 (37.3203, 28.6068) -> (37.8124, 31.3468)
  line L6 (37.8124, 31.3468) -> (35.2534, 30.2508)
  point P0 (0, 0)
  dimension "d40" = 3
  dimension "d44" = 4
  constraints: 8 end point, 5 point on circle, 5 tangent, 2 point on line, 1 centre point, 1 parallel, 1 perpendicular
  measures "d40" diameter of A0
  measures "d44" distance from line of L1 A0.centre
extrude "Extrusão5" cut sketch "Esboço6" against normal blind 10 contours L0 A0 L3 | A0 L0 | L0 A0 | L0 A1 L5 A0
equation "\"d7\" = d3"
